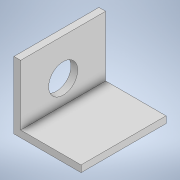
# Autodesk Inventor part: Big Motor Bracket
Saved by Autodesk Inventor 2022 (Build 260153000, 153)
## iProperties
Created: 2021-06-03
Part Number: Big Motor Bracket
Material: Generic
Document SubType Name: Modeling
Designer: jrcol
Density: 1 g/cm^3
Appearance: Default
Author: jrcol
Autodesk Inventor part; units mm, degrees
ref_plane "YZ Plane" through (0, 0, 0) normal (1, 0, 0) x (0, 1, 0)
ref_plane "XZ Plane" through (0, 0, 0) normal (0, 1, 0) x (-1, 0, 0)
ref_plane "XY Plane" through (0, 0, 0) normal (0, 0, 1) x (1, 0, 0)
sketch "Sketch1" plane through (0, 0, 0) normal (0, 1, 0) x (-1, 0, 0)
  line L0 (0, 0) -> (30, 0)
  line L1 (30, 0) -> (30, 38)
  line L2 (30, 38) -> (0, 38)
  line L3 (0, 38) -> (0, 0)
  dimension "d0" = 38
  dimension "d1" = 30
  constraints: 8 end point, 2 parallel, 1 horizontal, 1 perpendicular
  measures "d0" distance of L0.end L1.end
  measures "d1" distance of L1.end L2.end
extrude "Extrusion1" add sketch "Sketch1" along normal blind 3
sketch "Sketch2" plane through (0, 3, 0) normal (0, 1, 0) x (1, 0, 0)
  line L0 (-30, 0) -> (-30, -38) projected
  line L1 (0, 0) -> (-30, 0) projected
  line L2 (-30, -38) -> (-27, -38)
  line L3 (-27, -38) -> (-27, 0)
  line L4 (-27, 0) -> (-30, 0)
  line L5 (-30, 0) -> (-30, -38)
  dimension "d4" = 3
  constraints: 8 end point, 2 parallel, 1 horizontal, 1 perpendicular, 1 point on line
  measures "d4" distance of L0.end L2.end
extrude "Extrusion2" add sketch "Sketch2" along normal blind 27
sketch "Sketch3" plane through (-27, 3, 38) normal (1, 0, 0) x (0, 0, -1)
  circle A0 centre (19, 10.5) radius 6.5
  line L0 (38, 27) -> (0, 27) projected
  point P0 (38, -3)
  dimension "d7" = 13
  dimension "d8" = 16.5
  constraints: 1 centre point
  measures "d7" diameter of A0
  measures "d8" distance from line of L0 A0.centre
extrude "Extrusion3" cut sketch "Sketch3" against normal up to surface (3 mm away)
body "Solid1"
